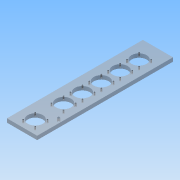
# Autodesk Inventor part: Tunel_LidWithFanHoles
Saved by Autodesk Inventor 2016 (Build 200138000, 138)
## iProperties
Created: 2014-10-15
Part Number: Tunel_LidWithFanHoles
Material: Polycarbonat, klar
Document SubType Name: Modeling
Designer: Gero Hofmann
Density: 1.2 g/cm^3
Appearance: Polycarbonat - klar
Author: Gero Hofmann
Autodesk Inventor part; units mm, degrees
ref_plane "YZ Plane" through (0, 0, 0) normal (1, 0, 0) x (0, 1, 0)
ref_plane "XZ Plane" through (0, 0, 0) normal (0, 1, 0) x (-1, 0, 0)
ref_plane "XY Plane" through (0, 0, 0) normal (0, 0, 1) x (1, 0, 0)
sketch "Skizze1" plane through (0, 0, 0) normal (0, 0, 1) x (1, 0, 0)
  line L0 (40, 180) -> (-40, 180)
  line L1 (-40, 180) -> (-40, -180)
  line L2 (-40, -180) -> (40, -180)
  line L3 (40, -180) -> (40, 180)
  line L4 (40, 180) -> (-40, -180) construction
  line L5 (-40, 180) -> (40, -180) construction
  point P0 (0, 0)
  dimension "d0" = 80
  dimension "d1" = 360
  constraints: 12 end point, 2 midpoint, 2 parallel, 1 horizontal, 1 perpendicular
  measures "d0" distance of L1.end L2.end
  measures "d1" distance of L0.end L1.end
extrude "Extrusion1" add sketch "Skizze1" along normal blind 10
hole "Bohrung3" at (27, -110, 10) direction (0, 0, -1) diameter 6 end through all
sketch "Skizze2" plane through (0, 0, 10) normal (0, 0, 1) x (1, 0, 0)
  line L0 (40, 180) -> (-40, 180) projected
  circle A0 centre (0, 130) radius 20
  point P0 (0, 0)
  dimension "d40" = 40
  dimension "d41" = 50
  constraints: 1 centre point
  measures "d40" diameter of A0
  measures "d41" distance from line of L0 A0.centre
extrude "Extrusion2" cut sketch "Skizze2" against normal blind 10
sketch "Skizze3" plane through (0, 0, 10) normal (0, 0, 1) x (1, 0, 0)
  circle A0 centre (0, 130) radius 20 projected
  line L0 (16, 114) -> (-16, 114)
  line L1 (-16, 114) -> (-16, 146)
  line L2 (-16, 146) -> (16, 146)
  line L3 (16, 146) -> (16, 114)
  line L4 (16, 114) -> (-16, 146) construction
  line L5 (-16, 114) -> (16, 146) construction
  dimension "d45" = 32
  constraints: 12 end point, 2 midpoint, 2 parallel, 2 perpendicular, 1 coincident, 1 horizontal
  measures "d45" distance of L1.end L2.end
hole "Bohrung4" at (16, 114, 10) at (-16, 114, 10) at (-16, 146, 10) at (16, 146, 10) direction (0, 0, -1) diameter 3.242 depth 8 tip angle 118 thread size "M4x0.7" class "6H" standard "ISO Metric profile"
pattern_linear "Rechteckige Anordnung3" count 5 spacing 50 along (0, -1, 0) of "Extrusion2", "Bohrung4"
pattern_linear "Rechteckige Anordnung4" count 2 spacing 275 along (0, -1, 0) of "Extrusion2", "Bohrung4"
